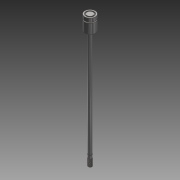
# Autodesk Inventor part: Rebuild Shooter NCDME075-0600 Rod
Saved by Autodesk Inventor 2014 SP1 (Build 180222100, 222)
## iProperties
Created: 2013-12-19
Part Number: Rebuild Shooter NCDME075-0600 Rod
Material: Stainless Steel
Document SubType Name: Modeling
Designer: Moses
Density: 8.08 g/cm^3
Appearance: Steel - Polished
Mass: 109.05 g
Surface Area: 67.6762 cm^2
Volume: 13.4963 cm^3
Author: Moses
Autodesk Inventor part; units mm, degrees
ref_plane "YZ Plane" through (0, 0, 0) normal (1, 0, 0) x (0, 1, 0)
ref_plane "XZ Plane" through (0, 0, 0) normal (0, 1, 0) x (-1, 0, 0)
ref_plane "XY Plane" through (0, 0, 0) normal (0, 0, 1) x (1, 0, 0)
sketch "Sketch1" plane through (0, 0, 0) normal (1, 0, 0) x (0, 1, 0)
  line L0 (0, 0) -> (0, 2.54)
  line L1 (0, 0) -> (235.6158, 0)
  line L2 (210.2158, 2.54) -> (210.2158, 3.175) construction
  line L3 (210.2158, 9.525) -> (227.6783, 9.525)
  line L4 (235.6158, 9.525) -> (235.6158, 7.1437)
  line L5 (12.7, 2.54) -> (12.7, 3.175)
  line L6 (12.7, 3.175) -> (18.415, 3.175)
  line L7 (19.05, 3.175) -> (19.05, 2.54)
  line L8 (19.05, 2.54) -> (18.415, 2.54)
  line L9 (18.415, 2.54) -> (18.415, 3.175)
  line L10 (210.2158, 7.1437) -> (211.0096, 7.1437)
  line L11 (210.2158, 5.5563) -> (211.0096, 5.5563)
  arc A0 (211.0096, 5.5563) -> (211.0096, 7.1437) centre (211.0096, 6.35) ccw
  line L12 (235.6158, 7.1437) -> (234.8221, 7.1437)
  line L13 (235.6158, 5.5563) -> (234.8221, 5.5563)
  arc A1 (234.8221, 7.1437) -> (234.8221, 5.5563) centre (234.8221, 6.35) ccw
  line L14 (234.8221, 6.35) -> (211.0096, 6.35) construction
  line L15 (227.6783, 9.525) -> (227.6783, 7.9375)
  line L16 (227.6783, 7.9375) -> (229.2658, 7.9375)
  line L17 (229.2658, 7.9375) -> (229.2658, 9.525)
  line L18 (229.2658, 9.525) -> (235.6158, 9.525)
  line L19 (227.6783, 9.525) -> (229.2658, 9.525)
  line L20 (19.05, 3.175) -> (210.2158, 3.175)
  line L21 (0, 2.54) -> (12.7, 2.54)
  line L22 (19.05, 2.54) -> (210.2158, 2.54) construction
  line L23 (12.7, 2.54) -> (18.415, 2.54) construction
  line L24 (210.2158, 3.175) -> (210.2158, 5.5563)
  line L25 (210.2158, 7.1437) -> (210.2158, 9.525)
  line L26 (210.2158, 5.5563) -> (210.2158, 7.1437) construction
  line L27 (235.6158, 7.1437) -> (235.6158, 5.5563) construction
  line L28 (235.6158, 5.5563) -> (235.6158, 0)
  dimension "d0" = 2.54
  dimension "d3" = 210.2158
  dimension "d4" = 25.4
  dimension "d5" = 9.525
  dimension "d22" = 0.635
  dimension "d23" = 12.7
  dimension "d27" = 0.635
  dimension "d28" = 5.715
  dimension "d32" = 1.5875
  dimension "d33" = 0.7937
  dimension "d35" = 12.7
  dimension "d36" = 1.5875
  dimension "d51" = 6.35
  dimension "d52" = 1.5875
  constraints: 58 end point, 16 horizontal, 11 vertical, 5 equal length, 4 point on circle, 3 point on line, 3 tangent, 2 centre point, 1 parallel
  measures "d0" distance of L0.end L0.start
  measures "d3" distance of L0.end L2.start
  measures "d4" distance of L4.start L3.start
  measures "d5" distance of L4.start L1.end
  measures "d22" distance of L5.start L5.end
  measures "d23" distance from line of L0.end L5
  measures "d27" distance of L6.end L7.start
  measures "d28" distance of L5.start L8.end
  measures "d32" distance of L10.start L11.start
  measures "d33" distance of L10.start L10.end
  measures "d35" diameter of L14.end L1
  measures "d36" distance of L4.end L13.start
  measures "d51" distance between parallel lines of L4 L17
  measures "d52" distance of L15.end L16.end
revolve "Revolution1" add sketch "Sketch1" angle 360 about axis through (0, 0, 0) along (0, 1, 0) contours L0 L21 L5 L6 L9 L8 L7 L20 L24 L11 A0 L10 L25 L3 L15 L16 L17 L18 L4 L12 A1 L13 L28 L1
sketch "Sketch4" plane through (0, 0, 0) normal (1, 0, 0) x (0, 1, 0)
  point P0 (0, 0)
sketch "Sketch5" plane through (0, 0, 0) normal (1, 0, 0) x (0, 1, 0)
  line L0 (0, 2.54) -> (12.7, 2.54) projected
  line L1 (0, 2.54) -> (-0.3666, 3.175)
  line L2 (-0.3666, 3.175) -> (-0.6206, 3.175)
  line L3 (-0.6206, 3.175) -> (-0.9872, 2.54)
  line L4 (-0.9872, 2.54) -> (0, 2.54)
  line L5 (0, -2.54) -> (0, 2.54) projected
  point P0 (0, 0)
  dimension "d37" = 0.254
  dimension "d38" = 60
  dimension "d39" = 0.635
  dimension "d53" = 0
  dimension "d54" = 0
  constraints: 8 end point, 2 horizontal, 1 equal length, 1 other
  measures "d37" distance of L1.end L2.end
  measures "d38" angle of L1 L3
  measures "d39" distance between parallel lines of L4 L2
  measures "d54" distance between parallel lines of L0 L4
coil "Coil2" sketch "Sketch5" operation add axis through (0, 6.35, 0) along (0, 1, 0) pitch 1.27 turns 11 hand right
sketch "Sketch6" plane through (0, 0, 0) normal (0, -1, 0) x (0.7652, 0, 0.6438)
  arc A0 (-1.6353, 1.9436) -> (1.6353, 1.9436) centre (0, 0) ccw projected
  circle A1 centre (0, 0) radius 2.54 projected
  circle A2 centre (0, 0) radius 6.35
  dimension "d48" = 12.7
  constraints: 1 centre point, 1 coincident
  measures "d48" diameter of A2
extrude "Extrusion3" cut sketch "Sketch6" along normal through all
equation "\"d52\" = d36"
body "Solid1"
